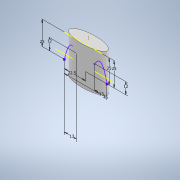
# Autodesk Inventor part: Practica 15
Saved by Autodesk Inventor 2020.2 (Build 242310000, 310)
## iProperties
Created: 2020-03-03
Part Number: Practica 15
Material: Genérico
Document SubType Name: Chapa
Designer: Luis Gallardo
Density: 1 g/cm^3
Sheet Metal Rule: Por defecto_mm
Appearance: Valor por defecto
Author: Luis Gallardo
Autodesk Inventor part; units mm, degrees
ref_plane "YZ Plane" through (0, 0, 0) normal (1, 0, 0) x (0, 1, 0)
ref_plane "XZ Plane" through (0, 0, 0) normal (0, 1, 0) x (-1, 0, 0)
ref_plane "XY Plane" through (0, 0, 0) normal (0, 0, 1) x (1, 0, 0)
sketch "Boceto1" plane through (0, 0, 0) normal (0, 1, 0) x (-1, 0, 0)
  ellipse E0 centre (0, 0) end of major axis (20, 0) minor radius 7
  line L0 (0, -7) -> (0, 7) construction
  line L1 (20, 0) -> (-20, 0) construction
  point P0 (0, 0)
  dimension "d1" = 7
  dimension "d11" = 40
  constraints: 4 end point, 3 midpoint, 1 coincident, 1 horizontal, 1 vertical, 6 other
  measures "d11" distance of L1.start L1.end
extrude "Extrusión1" add sketch "Boceto1" along normal blind 40
ref_plane "Plano de trabajo1" through (0, 20, 0) normal (0, 1, 0) x (1, 0, 0)
sketch "Boceto3" plane through (0, 20, 0) normal (0, 1, 0) x (1, 0, 0)
  line L0 (0, 0) -> (0, -5.552)
  ellipse E0 centre (0, 0) end of major axis (-20, 0) minor radius 7 projected
  constraints: 2 end point, 1 vertical, 1 other
ref_plane "Plano de trabajo3" through (0, 20, 5.552) normal (0, 0, 1) x (1, 0, 0)
sketch "Boceto4" plane through (0, 20, 5.552) normal (0, 0, 1) x (1, 0, 0)
  spline S0 degree 4 poles (-20.0856, -5) (-5.2067, 62.3041) (2.4144, -94.7389) (10.0356, 62.3041) (24.9144, -5) knots 0 0 0 0 0 1 1 1 1 1
  line L0 (-29.7165, 0) -> (34.5494, 0) projected
  line L1 (20, 20) -> (-20, 20) projected
  point P0 (0, -20)
  point P1 (-7.0856, 7)
  point P2 (1.8518, 0)
  point P3 (11.9144, 7)
  point P4 (2.4144, -5)
  dimension "d5" = 12
  dimension "d6" = 45
  dimension "d7" = 13
  dimension "d8" = 13
  dimension "d10" = 12
  dimension "d13" = 25
  dimension "d14" = 25
  dimension "d15" = 25
  dimension "d16" = 22.5
  constraints: 1 point on line, 5 other
  measures "d5" vertical distance of point (-20.086, -5) point (-7.086, 7)
  measures "d6" distance of point (24.914, -5) point (-20.086, -5)
  measures "d7" horizontal distance of point (-20.086, -5) point (-7.086, 7)
  measures "d8" horizontal distance of point (24.914, -5) point (11.914, 7)
  measures "d10" vertical distance of point (24.914, -5) point (11.914, 7)
  measures "d13" distance from line of L1 point (24.914, -5)
  measures "d14" distance from line of L1 point (-20.086, -5)
  measures "d15" distance from line of L1 point (2.414, -5)
  measures "d16" distance of point (-20.086, -5) point (2.414, -5)
equation "\"Radio_pliegue\" = Grosor"
equation "\"Anchura_desahogo_plegado\" = Grosor"
equation "\"Profundidad_desahogo_plegado\" = 0.5 * Grosor"
equation "\"Tamaño_destalonado\" = 4 * Grosor"
equation "\"Remanente_mínimo\" = 2 * Grosor"
equation "\"Radiodetransición\" = Radio_pliegue"
equation "\"Tamaño_de_radio_de_Jacobi\" = Radio_pliegue"
equation "\"TamañoSeparación\" = Grosor"
equation "\"Grosor\" = 0.5"
